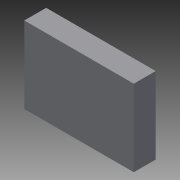
# Autodesk Inventor part: batt
Saved by Autodesk Inventor 2014 (Build 180170000, 170)
## iProperties
Created: 2013-09-12
Part Number: batt
Material: 一般
Document SubType Name: Modeling
Designer: koki
Density: 1 g/cm^3
Appearance: 既定
Author: koki
Autodesk Inventor part; units mm, degrees
ref_plane "YZ Plane" through (0, 0, 0) normal (1, 0, 0) x (0, 1, 0)
ref_plane "XZ Plane" through (0, 0, 0) normal (0, 1, 0) x (-1, 0, 0)
ref_plane "XY Plane" through (0, 0, 0) normal (0, 0, 1) x (1, 0, 0)
sketch "スケッチ1" plane through (0, 0, 0) normal (0, 1, 0) x (-1, 0, 0)
  line L0 (-19.4182, 10.0117) -> (-119.4182, 10.0117)
  line L1 (-119.4182, 10.0117) -> (-119.4182, -59.9883)
  line L2 (-119.4182, -59.9883) -> (-19.4182, -59.9883)
  line L3 (-19.4182, -59.9883) -> (-19.4182, 10.0117)
  point P0 (0, 0)
  dimension "d0" = 100
  dimension "d1" = 70
  constraints: 8 end point, 2 parallel, 1 horizontal, 1 perpendicular
  measures "d0" distance of L2.end L1.end
  measures "d1" distance of L1.end L0.end
extrude "押し出し1" add sketch "スケッチ1" along normal blind 20
